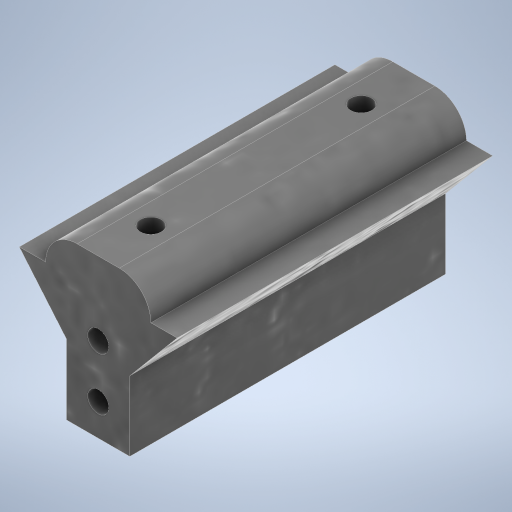
# Autodesk Inventor part: Foot_V1
Saved by Autodesk Inventor 2024 (Build 280153000, 153)
## iProperties
Created: 2024-06-05
Part Number: Foot_V1
Material: Generic
Document SubType Name: Modeling
Designer: Hemant
Density: 1 g/cm^3
Appearance: Fine Textured - Black
Author: Hemant
Autodesk Inventor part; units mm, degrees
ref_plane "YZ Plane" through (0, 0, 0) normal (1, 0, 0) x (0, 1, 0)
ref_plane "XZ Plane" through (0, 0, 0) normal (0, 1, 0) x (-1, 0, 0)
ref_plane "XY Plane" through (0, 0, 0) normal (0, 0, 1) x (1, 0, 0)
sketch "Sketch1" plane through (0, 0, 0) normal (0, 0, 1) x (1, 0, 0)
  line L0 (2, 7.5) -> (-2, 7.5)
  line L1 (-5, 4.5) -> (-5, -7.5)
  line L2 (-5, -7.5) -> (5, -7.5)
  line L3 (5, -7.5) -> (5, 4.5)
  line L4 (5, 7.5) -> (-5, -7.5) construction
  line L5 (-5, 7.5) -> (5, -7.5) construction
  arc A0 (-2, 7.5) -> (-5, 4.5) centre (-2, 4.5) ccw
  arc A1 (5, 4.5) -> (2, 7.5) centre (2, 4.5) ccw
  circle A2 centre (0, -4.5) radius 1
  circle A3 centre (0, 0.5) radius 1
  line L6 (-10.3044, 3.5) -> (10.8002, 3.5) construction
  line L7 (-3, -7.5) -> (-3, 3.5)
  line L8 (-3, 3.5) -> (-5, 3.5)
  line L9 (3, -7.5) -> (3, 3.5)
  line L10 (3, 3.5) -> (5, 3.5)
  point P0 (0, 0)
  point P1 (0, 7.5)
  dimension "d0" = 10
  dimension "d1" = 15
  dimension "d2" = 3
  dimension "d3" = 2
  dimension "d4" = 2
  dimension "d5" = 3
  dimension "d6" = 5
  dimension "d9" = 3
  dimension "d10" = 3
  dimension "d11" = 3
  constraints: 22 end point, 10 point on line, 4 centre point, 4 perpendicular, 4 point on circle, 4 tangent, 2 horizontal, 2 midpoint, 2 parallel, 2 vertical alignment, 1 equal radius, 1 vertical
  measures "d0" distance of L2.end L1.end
  measures "d1" distance of L1.end L5.start
  measures "d2" radius of A0
  measures "d3" diameter of A2
  measures "d4" diameter of A3
  measures "d5" distance from line of L2 A2.centre
  measures "d6" distance of A2.centre A3.centre
  measures "d9" distance from line of L6 A3.centre
  measures "d10" distance from line of L7 A2.centre
  measures "d11" distance from line of L9 A3.centre
extrude "Extrusion1" add sketch "Sketch1" along normal blind 30 contours A1 L3 L10 L9 L2 L7 L8 L1 A0 L0
chamfer "Chamfer1" distance 3.4641 angle 30 1 edges at (3, 3.5, 15) measured on face at (3, -3.8333, 10)
chamfer "Chamfer2" distance 3.4641 angle 30 1 edges at (-3, 3.5, 15) measured on face at (-3, -0.1667, 10)
sketch "Sketch2" plane through (-2, 7.5, 0) normal (0, 1, 0) x (1, 0, 0)
  circle A0 centre (2, -25) radius 1
  circle A1 centre (2, -5) radius 1
  line L0 (4, 0) -> (0, 0) projected
  line L1 (4, -30) -> (0, -30) projected
  point P0 (2, 0)
  point P1 (2, 0)
  point P2 (2, 0)
  dimension "d19" = 2
  dimension "d20" = 2
  dimension "d21" = 5
  dimension "d22" = 5
  constraints: 2 centre point, 2 midpoint, 2 vertical alignment
  measures "d19" diameter of A0
  measures "d20" diameter of A1
  measures "d21" distance of point (2, 0) A1.centre
  measures "d22" distance from line of L1 A0.centre
extrude "Extrusion2" cut sketch "Sketch2" against normal blind 3
sketch "Sketch3" plane through (0, 0, 30) normal (0, 0, 1) x (1, 0, 0)
  line L0 (-3, -7.5) -> (3, -7.5) projected
  line L1 (3, -7.5) -> (7.5, -7.5) construction
  line L2 (7.5, -7.5) -> (7.5, 4.5) construction
  line L3 (7.5, 4.5) -> (5, 4.5) construction
  line L4 (3, 4.5) -> (3, -7.5) construction
  line L5 (7.5, 4.5) -> (3, -0.8629)
  line L6 (7.5, 4.5) -> (13.864, 4.5) construction
  line L7 (7.5, 4.5) -> (5, 4.5)
  line L8 (5, 3.5) -> (3, 0.0359) projected
  line L9 (5, 3.5) -> (5, 4.5) projected
  line L10 (3, -7.5) -> (3, 0.0359) projected
  point P0 (0, 0)
  dimension "d25" = 4.5
  dimension "d26" = 12
  dimension "d27" = 130
  constraints: 14 end point, 2 horizontal, 2 parallel, 2 point on line, 1 perpendicular
  measures "d25" distance of L4.start L2.end
  measures "d26" distance of L2.end L1.end
  measures "d27" angle of L5 L6
extrude "Extrusion3" add sketch "Sketch3" against normal up to surface (30 mm away)
mirror "Mirror2" about plane through (0, 0, 0) normal (1, 0, 0) of "Extrusion3"
body "Solid1"
